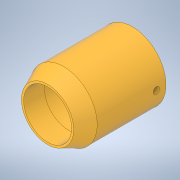
# Autodesk Inventor part: Nikon-Objective-Insulation_singe_cable_grooves_v2
Saved by Autodesk Inventor 2020 (Build 240168000, 168)
## iProperties
Created: 2018-11-08
Part Number: Nikon-Objective-Insulation_singe_cable_grooves_v2
Material: ABS Plastic
Document SubType Name: Modeling
Designer: rainer
Density: 1.06 g/cm^3
Appearance: Smooth - White
Author: rainer
Autodesk Inventor part; units mm, degrees
ref_plane "XZ Plane" through (0, 0, 0) normal (0, 1, 0) x (-1, 0, 0)
ref_plane "XY Plane" through (0, 0, 0) normal (0, 0, 1) x (1, 0, 0)
sketch "Sketch1" plane through (0, 0, 0) normal (0, 0, 1) x (1, 0, 0)
  circle A0 centre (0, 0) radius 15
  circle A1 centre (0, 0) radius 21
  dimension "d0" = 30
  dimension "d1" = 42
  constraints: 2 centre point, 2 coincident
  measures "d0" diameter of A0
  measures "d1" diameter of A1
extrude "Extrusion1" add sketch "Sketch1" along normal blind 53
sketch "Sketch2" plane through (0, 0, 0) normal (0, 0, -1) x (-1, 0, 0)
  circle A0 centre (0, 0) radius 17.5
  circle A1 centre (0, 0) radius 21
  dimension "d4" = 35
  dimension "d5" = 42
  constraints: 2 centre point, 2 coincident
  measures "d4" diameter of A0
  measures "d5" diameter of A1
extrude "Extrusion2" add sketch "Sketch2" along normal blind 5
chamfer "Chamfer2" distance 10 angle 25 1 edges at (-21, 0, 53)
thicken "Thicken1" operation add thickness 5 both sides no extend neighbours yes toward (0, 0, 1) faces at (-19.46042, -3.071218, -5)
sketch "Sketch3" plane through (0, 0, 0) normal (0, 0, -1) x (-1, 0, 0)
  circle A0 centre (0, 0) radius 15.25
  dimension "d16" = 30.5
  constraints: 1 centre point, 1 coincident
  measures "d16" diameter of A0
extrude "Extrusion3" cut sketch "Sketch3" against normal blind 40
sketch "Sketch4" plane through (0, 0, 0) normal (0, 0, -1) x (-1, 0, 0)
  circle A0 centre (0, 0) radius 15.25 projected
  circle A1 centre (-15.25, 0) radius 2
  dimension "d19" = 4
  constraints: 1 centre point, 1 horizontal alignment, 1 other
  measures "d19" diameter of A1
extrude "Extrusion4" cut sketch "Sketch4" against normal blind 40 contours A1 A0 | A0 A1 picked at (-14.573606, 0) picked at (-15.90694, 0)
sketch "Sketch5" plane through (0, 0, 40) normal (0, 0, -1) x (-1, 0, 0)
  circle A0 centre (0, 0) radius 15 projected
  circle A1 centre (-15, 0) radius 1.5
  point P0 (-14.925, -1.498124)
  point P1 (-14.925, 1.498124)
  dimension "d22" = 3
  constraints: 1 centre point, 2 other
  measures "d22" diameter of A1
extrude "Extrusion5" cut sketch "Sketch5" against normal blind 5 contours A0 A1 picked at (-15.490559, 0.062178)
ref_plane "Work Plane1" through (21, 0, 0) normal (1, 0, 0) x (0, 1, 0)
sketch "Sketch6" plane through (21, 0, 0) normal (1, 0, 0) x (0, 1, 0)
  circle A0 centre (0, 6) radius 2
  line L0 (-21, 0) -> (21, 0) projected
  point P0 (0, 0)
  dimension "d26" = 4
  dimension "d27" = 6
  constraints: 1 centre point
  measures "d26" diameter of A0
  measures "d27" distance from line of L0 A0.centre
extrude "Extrusion6" cut sketch "Sketch6" against normal blind 10
sketch "Sketch7" plane through (0, 0, 0) normal (0, 0, -1) x (-1, 0, 0)
  line L0 (0, 0) -> (-13.610618, 10.59781)
  line L1 (0, 0) -> (-16.169661, 6.008708)
  arc A0 (-15.118852, 1.995695) -> (-15.118852, -1.995695) centre (-15.25, 0) ccw
  arc A1 (-13.610618, 10.59781) -> (-17.25, 0) centre (0, 0) ccw
  arc A2 (-15.118852, -1.995695) -> (-15.118852, 1.995695) centre (0, 0) ccw
  arc A3 (-12.032576, 9.369078) -> (-15.25, 0) centre (0, 0) ccw
  circle A4 centre (-13.15738, 7.710113) radius 2
  point P0 (-14.882938, 8.721276)
  point P1 (-12.035243, 9.365652)
  dimension "d30" = 17.25
  dimension "d31" = 17.25
  dimension "d38" = 4
  constraints: 8 point on circle, 4 end point, 3 centre point, 1 point on line, 1 tangent
  measures "d30" distance of L0.start L0.end
  measures "d31" distance of L1.start L1.end
  measures "d38" diameter of A4
extrude "Extrusion7" cut sketch "Sketch7" against normal blind 40 contours A2 A4 | A4 A2 L1 A1 | A1 L1 A2 A0 picked at (-13.724174, 8.042249)
fillet "Fillet1" radius 1.9999 2 edges at (16.6477, 4.5184, 40) (16.6171, -1.4598, 40)
body "Solid1"
